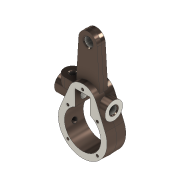
# Autodesk Inventor part: Part002.Lever
Saved by Autodesk Inventor 2022.2 (Build 262287010, 287A)
## iProperties
Created: 2022-11-28
Part Number: Part002.Lever
Material: Steel, Carbon
Document SubType Name: Modeling
Designer: User
Mass: 1149.81 g
Surface Area: 383.206 cm^2
Volume: 146.473 cm^3
Density: 7.85 g/cm^3
Appearance: Semi-Polished
Author: User
Autodesk Inventor part; units mm, degrees
ref_plane "XY Plane" through (0, 0, 0) normal (0, 0, 1) x (1, 0, 0)
sketch "Sketch1" plane through (0, 0, 0) normal (0, 0, 1) x (1, 0, 0)
  arc A0 (-38.7386, 16.2273) -> (38.7386, 16.2273) centre (0, 0) ccw
  line L0 (-38.7386, 16.2273) -> (-23.0587, 53.6591)
  arc A1 (23.0587, 53.6591) -> (-23.0587, 53.6591) centre (0, 44) ccw
  line L1 (23.0587, 53.6591) -> (38.7386, 16.2273)
  dimension "d0" = 84
  dimension "d2" = 44
  dimension "d3" = 25
  constraints: 4 end point, 4 point on circle, 4 tangent, 2 centre point, 1 coincident, 1 vertical alignment
  measures "d0" diameter of A0
  measures "d2" distance of A0.centre A1.centre
  measures "d3" radius of A1
extrude "Extrusion1" add sketch "Sketch1" along normal mid plane 32 draft -2
sketch "Sketch2" plane through (0, 0, 0) normal (0, 0, 1) x (1, 0, 0)
  line L0 (-20.9841, 44) -> (20.9841, 44)
  arc A0 (15.9702, 125.9768) -> (-15.9702, 125.9768) centre (0, 125) ccw
  arc A1 (22.5433, 53.4432) -> (-22.5433, 53.4432) centre (0, 44) ccw construction
  line L1 (-15.9702, 125.9768) -> (-20.9841, 44)
  line L2 (15.9702, 125.9768) -> (20.9841, 44)
  point P0 (0, 0)
  dimension "d6" = 16
  dimension "d7" = 7
  dimension "d8" = 125
  constraints: 6 end point, 2 point on circle, 2 tangent, 1 centre point, 1 coincident, 1 horizontal, 1 midpoint, 1 vertical alignment
  measures "d6" radius of A0
  measures "d7" angle of L2 L1
  measures "d8" distance of point (0, 0) A0.centre
extrude "Extrusion2" add sketch "Sketch2" along normal mid plane 14 draft -2
ref_plane "Work Plane2" through (37, 0, 0) normal (1, 0, 0) x (0, 1, 0)
sketch "Sketch3" plane through (37, 0, 0) normal (1, 0, 0) x (0, 1, 0)
  circle A0 centre (39.5, 0) radius 15
  line L0 (16.0114, 16) -> (16.0114, 16) projected
  line L1 (16.2273, 0) -> (16.0114, 16) projected
  line L2 (16.2273, 0) -> (16.2273, 0) projected
  line L3 (16.2273, 0) -> (16.0114, 16) projected
  line L4 (53.4432, 16) -> (16.0114, 16) projected
  line L5 (16.2273, 0) -> (16.0114, 16) projected
  line L6 (16.2273, 0) -> (53.6591, 0) projected
  line L7 (53.6591, 0) -> (53.4432, 16) projected
  line L8 (16.0114, -16) -> (-41.4413, -16) projected
  line L9 (16.0114, -16) -> (53.4432, -16) projected
  line L10 (53.6591, 0) -> (53.4432, -16) projected
  line L11 (16.2273, 0) -> (53.6591, 0) projected
  line L12 (16.2273, 0) -> (16.0114, -16) projected
  point P0 (0, 0)
  dimension "d12" = 30
  dimension "d13" = 39.5
  constraints: 1 centre point, 1 horizontal alignment
  measures "d12" diameter of A0
  measures "d13" distance of point (0, 0) A0.centre
extrude "Extrusion3" add sketch "Sketch3" against normal blind 86 contours A0 L10 L7 | L7 L6 A0 | A0 L6 L10
sketch "Sketch4" plane through (0, 0, 16) normal (0, 0, 1) x (1, 0, 0)
  line L0 (-38.2232, 16.0114) -> (-22.5433, 53.4432) projected
  arc A0 (-38.2232, 16.0114) -> (38.2232, 16.0114) centre (0, 0) ccw projected
  line L1 (22.5433, 53.4432) -> (38.2232, 16.0114) projected
  arc A1 (22.5433, 53.4432) -> (-22.5433, 53.4432) centre (0, 44) ccw projected
  circle A2 centre (0, 0) radius 31
  line L2 (-13, 0) -> (13, 0)
  line L3 (13, 0) -> (13, 55)
  line L4 (13, 55) -> (-13, 55)
  line L5 (-13, 55) -> (-13, 0)
  point P0 (-13, 28.1425)
  point P1 (13, 28.1425)
  dimension "d16" = 62
  dimension "d17" = 26
  dimension "d18" = 55
  constraints: 8 end point, 2 coincident, 2 parallel, 1 centre point, 1 horizontal, 1 midpoint, 1 perpendicular
  measures "d16" diameter of A2
  measures "d17" distance between parallel lines of L3 L5
  measures "d18" distance between parallel lines of L2 L4
extrude "Extrusion4" cut sketch "Sketch4" against normal through all contours A2 L5 L2 L3 | L3 L2 L5 A2 | A2 L5 L4 L3
fillet "Fillet1" radius 1 2 edges at (-13, 55, 0) (13, 55, 0)
ref_plane "Work Plane3" through (0, 60.5, 0) normal (0, 1, 0) x (-1, 0, 0)
sketch "Sketch5" plane through (0, 60.5, 0) normal (0, 1, 0) x (-1, 0, 0)
  line L0 (13, 16) -> (13, -16) projected
  line L1 (13, -14) -> (33, -14)
  arc A0 (33, -14) -> (33, 14) centre (33, 0) ccw
  line L2 (33, 14) -> (13, 14)
  line L3 (13, 14) -> (13, -14)
  point P0 (0, 0)
  point P1 (13, 0)
  dimension "d23" = 33
  dimension "d24" = 14
  constraints: 6 end point, 2 midpoint, 2 point on circle, 1 centre point, 1 horizontal, 1 horizontal alignment, 1 parallel, 1 perpendicular, 1 tangent
  measures "d23" distance of point (0, 0) A0.centre
  measures "d24" radius of A0
extrude "Extrusion5" add sketch "Sketch5" against normal up to surface round surface about axis through (37, 39.5, 0) along (-1, 0, 0) radius 15 far side no
sketch "Sketch6" plane through (37, 39.5, 0) normal (1, 0, 0) x (0, 0, -1)
  circle A0 centre (0, 0) radius 15 projected
  point P0 (0, -39.5)
  constraints: 1 coincident
hole "Hole1" at (37, 39.5, 0) direction (-1, 0, 0) diameter 13 end through all
sketch "Sketch7" plane through (-49, 39.5, 0) normal (-1, 0, 0) x (0, 0, 1)
  circle A0 centre (0, 0) radius 15 projected
  point P0 (0, -39.5)
  constraints: 1 coincident
hole "Hole2" at (-49, 39.5, 0) direction (1, 0, 0) diameter 13.8 depth 36
sketch "Sketch8" plane through (0, 60.5, 0) normal (0, 1, 0) x (1, 0, 0)
  arc A0 (-33, 14) -> (-33, -14) centre (-33, 0) ccw projected
  point P0 (0, 0)
  constraints: 1 coincident
hole "Hole3" at (-33, 60.5, 0) direction (0, -1, 0) diameter 8.9175 end up to surface thread size "M10x1" class "6H" standard "ISO Metric profile"
sketch "Sketch9" plane through (0, 0, 7) normal (0, 0, 1) x (1, 0, 0)
  arc A0 (15.7262, 125.9619) -> (-15.7262, 125.9619) centre (0, 125) ccw projected
  point P0 (0, 0)
  constraints: 1 coincident
hole "Hole4" at (0, 125, 7) direction (0, 0, -1) diameter 15 end through all
sketch "Sketch10" plane through (0, 0, 16) normal (0, 0, 1) x (1, 0, 0)
  line L0 (0, 0) -> (-25.1023, 25.1023) construction
  line L1 (-67.2, 0) -> (60.2, 0) construction
  line L2 (-25.1023, 25.1023) -> (0, 0)
  line L3 (0, 0) -> (-25.1023, -25.1023) construction
  line L4 (0, 0) -> (25.1023, -25.1023) construction
  line L5 (0, 0) -> (25.1023, 25.1023) construction
  point P0 (0, 60)
  dimension "d55" = 45
  dimension "d56" = 35.5
  dimension "d57" = 60
  dimension "d60" = 360
  constraints: 10 end point, 4 point on line, 2 coincident, 1 vertical alignment, 15 other
  measures "d55" angle of L1 L0
  measures "d56" distance of L0.start L0.end
  measures "d57" distance of L0.start point (0, 60)
hole "Hole5" at (0, 60, 16) at (-25.1023, 25.1023, 16) at (-25.1023, -25.1023, 16) at (25.1023, -25.1023, 16) at (25.1023, 25.1023, 16) direction (0, 0, -1) diameter 4.3 end through all
sketch "Sketch11" plane through (0, 0, 0) normal (0, 0, 1) x (1, 0, 0)
  line L0 (0, 0) -> (-71.1948, -19.0766)
  line L1 (-95.6168, 0) -> (64.9361, 0) projected
  dimension "d69" = 15
  constraints: 2 end point
  measures "d69" angle of L1 L0
hole "Hole6" at (-40.5689, -10.8704, 0) direction (0.9659258, 0.258819, 0) diameter 8.9175 end up to surface thread size "M10x1" class "6H" standard "ISO Metric profile"
chamfer "Chamfer1" distance 1.5 angle 45 5 edges at (0, 132.5, -7) (0, 132.5, 7) (-49, 39.5, -6.9) (-33, 60.5, -4.4587) (37, 39.5, 6.5)
body "Solid1"
